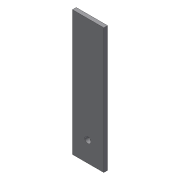
# Autodesk Inventor part: UPPER_LEG_BASE
Saved by Autodesk Inventor 2019.4 (Build 234330000, 330)
## iProperties
Created: 2019-12-01
Part Number: UPPER_LEG_BASE
Material: 一般
Document SubType Name: Modeling
Designer: y6tada
Density: 1 g/cm^3
Appearance: 既定
Author: y6tada
Autodesk Inventor part; units mm, degrees
ref_plane "YZ Plane" through (0, 0, 0) normal (1, 0, 0) x (0, 1, 0)
ref_plane "XZ Plane" through (0, 0, 0) normal (0, 1, 0) x (-1, 0, 0)
ref_plane "XY Plane" through (0, 0, 0) normal (0, 0, 1) x (1, 0, 0)
sketch "スケッチ1" plane through (0, 0, 0) normal (0, 0, 1) x (1, 0, 0)
  circle A0 centre (0, 0) radius 1.5
  circle A1 centre (13.5, 33.5) radius 1.25 construction
  circle A2 centre (13.5, 85.5) radius 1.25 construction
  circle A3 centre (-13.5, 85.5) radius 1.25 construction
  circle A4 centre (-13.5, 33.5) radius 1.25 construction
  circle A5 centre (0, 75) radius 1.5 construction
  circle A6 centre (0, 75) radius 13
  line L0 (16.884, 32.6064) -> (7.7349, -2.0424)
  line L1 (-7.7349, -2.0424) -> (-16.884, 32.6064)
  line L2 (-17, 33.5) -> (-17, 85.5)
  line L3 (-15.9749, 87.9749) -> (-8, 95.9497)
  line L4 (-8, 95.9497) -> (-8, 125)
  line L5 (8, 125) -> (8, 95.9497)
  line L6 (8, 95.9497) -> (15.9749, 87.9749)
  line L7 (17, 85.5) -> (17, 33.5)
  arc A7 (16.884, 32.6064) -> (17, 33.5) centre (13.5, 33.5) ccw
  arc A8 (17, 85.5) -> (15.9749, 87.9749) centre (13.5, 85.5) ccw
  arc A9 (-15.9749, 87.9749) -> (-17, 85.5) centre (-13.5, 85.5) ccw
  arc A10 (-17, 33.5) -> (-16.884, 32.6064) centre (-13.5, 33.5) ccw
  arc A11 (-7.7349, -2.0424) -> (7.7349, -2.0424) centre (0, 0) ccw
  line L8 (0, 0) -> (0, 152.1421) construction
  arc A12 (8, 125) -> (-8, 125) centre (0, 125) ccw
  point P0 (0, 113)
  dimension "d2" = 3
  dimension "d3" = 26
  dimension "d4" = 3.5
  dimension "d5" = 8
  dimension "d6" = 125
  dimension "d7" = 16
  dimension "d8" = 45
  dimension "d9" = 45
  dimension "d10" = 38
  constraints: 18 end point, 12 point on circle, 12 tangent, 8 centre point, 7 coincident, 5 concentric, 4 vertical, 3 equal radius, 2 point on line, 1 parallel
  measures "d2" diameter of A0
  measures "d3" diameter of A6
  measures "d4" radius of A7
  measures "d5" radius of A11
  measures "d6" distance of point (0, 0) A12.centre
  measures "d7" distance between parallel lines of L4 L5
  measures "d8" angle of L7 L6
  measures "d9" angle of L2 L3
  measures "d10" distance of A5.centre point (0, 113)
extrude "押し出し1" add sketch "スケッチ1" along normal blind 2
hole "穴2" at (0, 125, 0) direction (0, 0, 1) diameter 8 end through all
hole "穴3" at (0, 113, 0) direction (0, 0, 1) diameter 6 end through all
fillet "フィレット1" radius 6.5 2 edges at (-8, 95.9497, 1) (8, 95.9497, 1)
sketch "スケッチ2" plane through (0, 0, 2) normal (0, 0, 1) x (1, 0, 0)
  arc A0 (17, 85.5) -> (15.9749, 87.9749) centre (13.5, 85.5) ccw construction
  arc A1 (-15.9749, 87.9749) -> (-17, 85.5) centre (-13.5, 85.5) ccw construction
  arc A2 (-17, 33.5) -> (-16.884, 32.6064) centre (-13.5, 33.5) ccw construction
  arc A3 (16.884, 32.6064) -> (17, 33.5) centre (13.5, 33.5) ccw construction
  point P0 (0, 0)
  constraints: 4 coincident
hole "穴4" at (13.5, 85.5, 2) at (-13.5, 85.5, 2) at (-13.5, 33.5, 2) at (13.5, 33.5, 2) direction (0, 0, -1) diameter 2.6 end through all countersink diameter 5.5 countersink angle 90 clearance for "Countersunk Flat Head Screw ISO 2009/7046" size "M2.5" standard "ISO"
